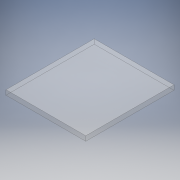
# Autodesk Inventor part: Frente-inferior-E-D
Saved by Autodesk Inventor 2017 (Build 210142000, 142)
## iProperties
Created: 2016-08-19
Part Number: Frente-inferior-E-D
Material: Polycarbonate, Clear
Document SubType Name: Modeling
Designer: Alunos
Density: 1.2 g/cm^3
Appearance: Polycarbonate - Clear
Author: Alunos
Autodesk Inventor part; units mm, degrees
ref_plane "YZ Plane" through (0, 0, 0) normal (1, 0, 0) x (0, 1, 0)
ref_plane "XZ Plane" through (0, 0, 0) normal (0, 1, 0) x (-1, 0, 0)
ref_plane "XY Plane" through (0, 0, 0) normal (0, 0, 1) x (1, 0, 0)
sketch "Sketch1" plane through (0, 0, 0) normal (0, 0, 1) x (1, 0, 0)
  line L0 (0, 0) -> (335, 0)
  line L1 (335, 0) -> (335, 130)
  line L2 (335, 130) -> (0, 130)
  line L3 (0, 130) -> (0, 0)
  dimension "d0" = 335
  dimension "d1" = 130
  constraints: 8 end point, 2 parallel, 1 horizontal, 1 perpendicular
  measures "d0" distance of L2.end L1.end
  measures "d1" distance of L1.end L0.end
extrude "Extrusion1" add sketch "Sketch1" along normal blind 7
sketch "Sketch2" plane through (0, 0, 7) normal (0, 0, 1) x (1, 0, 0)
  line L0 (0, 0) -> (335, 0) projected
  line L1 (0, 0) -> (127.5, 0)
  line L2 (127.5, 0) -> (207.5, 0)
  line L3 (207.5, 0) -> (335, 0)
  line L4 (335, 130) -> (0, 130) projected
  line L5 (0, 0) -> (167.5, 0)
  line L6 (167.5, 0) -> (117.5, 0)
  line L7 (117.5, 0) -> (217.5, 0)
  line L8 (217.5, 0) -> (217.5, 130)
  line L9 (117.5, 0) -> (117.5, 130)
  line L10 (117.5, 0) -> (0, 0)
  line L11 (217.5, 0) -> (335, 0)
  dimension "d7" = 100
  constraints: 20 end point, 6 point on line, 3 collinear, 2 perpendicular, 1 midpoint
  measures "d7" distance of L6.end L7.end
extrude "Extrusion2" cut sketch "Sketch2" against normal blind 10
sketch "Sketch3" plane through (0, 0, 7) normal (0, 0, 1) x (1, 0, 0)
  line L0 (335, 130) -> (217.5, 130) projected
  line L1 (335, 0) -> (335, 130) projected
  line L2 (217.5, 130) -> (335, 130)
  line L3 (335, 130) -> (335, 0)
  line L4 (335, 0) -> (217.5, 0)
  line L5 (217.5, 0) -> (217.5, 130)
  point P0 (0, 0)
  constraints: 8 end point, 2 parallel, 1 horizontal, 1 perpendicular
extrude "Extrusion3" cut sketch "Sketch3" against normal blind 10
body "Solid1"
